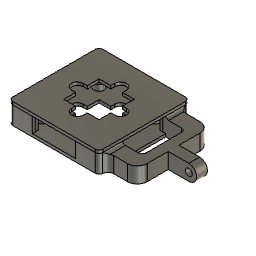
ArduCam Case v4 (Autodesk Fusion 360 design; units mm, degrees)
Autodesk Fusion 360 part; units mm, degrees
sketch "Base" plane through (0, 0, 0) normal (0, 0, 1) x (1, 0, 0)
  circle A0 centre (14.4, -14.4) radius 1.5
  circle A1 centre (-14.4, -14.4) radius 1.5
  circle A2 centre (-14.4, 14.4) radius 1.5
  circle A3 centre (14.4, 14.4) radius 1.5
  line L0 (18, 20) -> (-18, 20)
  line L1 (-20, 18) -> (-20, -18)
  line L2 (-18, -20) -> (18, -20)
  line L3 (20, -18) -> (20, 18)
  line L4 (19.5, -21.5) -> (-19.5, -21.5)
  line L5 (-21.5, -19.5) -> (-21.5, 19.5)
  line L6 (-19.5, 21.5) -> (19.5, 21.5)
  line L7 (21.5, -19.5) -> (21.5, 19.5)
  line L8 (21, 23) -> (-21, 23)
  line L9 (-23, 21) -> (-23, -21)
  line L10 (-21, -23) -> (21, -23)
  line L11 (23, 21) -> (23, -21)
  arc A4 (-18, 20) -> (-20, 18) centre (-18, 18) ccw
  arc A5 (-20, -18) -> (-18, -20) centre (-18, -18) ccw
  arc A6 (18, -20) -> (20, -18) centre (18, -18) ccw
  arc A7 (20, 18) -> (18, 20) centre (18, 18) ccw
  arc A8 (-19.5, 21.5) -> (-21.5, 19.5) centre (-19.5, 19.5) ccw
  arc A9 (-21.5, -19.5) -> (-19.5, -21.5) centre (-19.5, -19.5) ccw
  arc A10 (19.5, -21.5) -> (21.5, -19.5) centre (19.5, -19.5) ccw
  arc A11 (21.5, 19.5) -> (19.5, 21.5) centre (19.5, 19.5) ccw
  arc A12 (-21, 23) -> (-23, 21) centre (-21, 21) ccw
  arc A13 (-23, -21) -> (-21, -23) centre (-21, -21) ccw
  arc A14 (21, -23) -> (23, -21) centre (21, -21) ccw
  arc A15 (23, 21) -> (21, 23) centre (21, 21) ccw
  line L12 (9, -9) -> (-9, 9) construction
  line L13 (-9, -9) -> (9, 9) construction
  line L14 (9, 0) -> (11, 0)
  arc A16 (11, -3) -> (11, 3) centre (11, 0) ccw
  arc A17 (-3, -11) -> (3, -11) centre (0, -11) ccw
  arc A18 (-11, 3) -> (-11, -3) centre (-11, 0) ccw
  arc A19 (3, 11) -> (-3, 11) centre (0, 11) ccw
  line L15 (-9, 9) -> (-3, 9)
  line L16 (-3, 11) -> (-3, 9)
  line L17 (-9, 9) -> (-9, 3)
  line L18 (-9, 3) -> (-11, 3)
  line L19 (-11, -3) -> (-9, -3)
  line L20 (-9, -3) -> (-9, -9)
  line L21 (-9, -9) -> (-3, -9)
  line L22 (-3, -9) -> (-3, -11)
  line L23 (3, -11) -> (3, -9)
  line L24 (9, -3) -> (11, -3)
  line L25 (11, 3) -> (9, 3)
  line L26 (9, 3) -> (9, 9)
  line L27 (3, 9) -> (3, 11)
  line L28 (3, 9) -> (9, 9)
  line L29 (9, -9) -> (3, -9)
  line L30 (9, -9) -> (9, -3)
  circle A20 centre (14.4, 14.4) radius 2.5
  circle A21 centre (-14.4, 14.4) radius 2.5
  circle A22 centre (-14.4, -14.4) radius 2.5
  circle A23 centre (14.4, -14.4) radius 2.5
  line L31 (-23, -11) -> (-20, -11)
  line L32 (-20, 11) -> (-23, 11)
  line L33 (20, 11) -> (23, 11)
  line L34 (20, -11) -> (23, -11)
  line L35 (-11, 20) -> (-11, 23)
  line L36 (11, 20) -> (11, 23)
  line L37 (11, -20) -> (11, -23)
  line L38 (-11, -20) -> (-11, -23)
  circle A24 centre (-14.4, -14.4) radius 1.4
  circle A25 centre (14.4, -14.4) radius 1.4
  circle A26 centre (14.4, 14.4) radius 1.4
  circle A27 centre (-14.4, 14.4) radius 1.4
  point P0 (21.5, -21.5)
  point P1 (-21.5, -21.5)
  point P2 (-21.5, 21.5)
  point P3 (21.5, 21.5)
  dimension "d3" = 28.8
  dimension "d4" = 28.8
  dimension "d5" = 28.8
  dimension "d6" = 3
  dimension "d7" = 3
  dimension "d8" = 3
  dimension "d9" = 3
  dimension "d10" = 43
  dimension "d11" = 43
  dimension "d12" = 43
  dimension "d13" = 2
  dimension "d14" = 2
  dimension "d15" = 2
  dimension "d16" = 5
  dimension "d17" = 5
  dimension "d18" = 5
  dimension "d19" = 5
  dimension "d71" = 2.8
  dimension "d72" = 2.8
  dimension "d73" = 2.8
  dimension "d74" = 2.8
  constraint perpendicular L0 L1
  constraint perpendicular L1 L2
  constraint perpendicular L0 L3
  constraint perpendicular L4 L5
  constraint perpendicular L5 L6
  constraint perpendicular L5 L8
  constraint perpendicular L8 L9
  constraint perpendicular L9 L10
  constraint perpendicular L10 L11
  constraint tangent L0 A4
  constraint tangent L1 A4
  constraint tangent L1 A5
  constraint tangent L2 A5
  constraint equal A4 A5
  constraint tangent L2 A6
  constraint tangent L3 A6
  constraint equal A4 A6
  constraint tangent L0 A7
  constraint tangent L3 A7
  constraint equal A4 A7
  constraint coincident P2 L5
  constraint coincident P2 L6
  constraint tangent L5 A8
  constraint tangent L6 A8
  constraint coincident P1 L4
  constraint coincident P1 L5
  constraint tangent L4 A9
  constraint tangent L5 A9
  constraint equal A8 A9
  constraint coincident P0 L4
  constraint coincident P0 L7
  constraint tangent L4 A10
  constraint tangent L7 A10
  constraint equal A8 A10
  constraint coincident P3 L6
  constraint coincident P3 L7
  constraint tangent L6 A11
  constraint tangent L7 A11
  constraint equal A8 A11
  constraint tangent L8 A12
  constraint tangent L9 A12
  constraint tangent L9 A13
  constraint tangent L10 A13
  constraint equal A12 A13
  constraint tangent L10 A14
  constraint tangent L11 A14
  constraint equal A12 A14
  constraint tangent L8 A15
  constraint tangent L11 A15
  constraint equal A12 A15
  constraint coincident L12 origin
  constraint coincident L13 origin
  constraint coincident L14.end A16.centre
  constraint tangent A19 L16
  constraint tangent A18 L18
  constraint tangent A18 L19
  constraint tangent A17 L22
  constraint tangent A17 L23
  constraint tangent A16 L24
  constraint tangent A16 L25
  constraint tangent A19 L27
  constraint perpendicular L27 L28
  constraint perpendicular L23 L29
  constraint perpendicular L29 L30
  constraint concentric A3 A20
  constraint concentric A2 A21
  constraint concentric A1 A22
  constraint concentric A0 A23
  constraint coincident L9 L31.start
  constraint coincident L1 L31.end
  constraint perpendicular L1 L31
  constraint coincident L1 L32.start
  constraint coincident L9 L32.end
  constraint perpendicular L9 L32
  constraint coincident L3 L33.start
  constraint coincident L11 L33.end
  constraint perpendicular L11 L33
  constraint coincident L3 L34.start
  constraint coincident L11 L34.end
  constraint perpendicular L11 L34
  constraint coincident L0 L35.start
  constraint coincident L8 L35.end
  constraint perpendicular L8 L35
  constraint coincident L0 L36.start
  constraint coincident L8 L36.end
  constraint perpendicular L8 L36
  constraint coincident L2 L37.start
  constraint coincident L10 L37.end
  constraint perpendicular L10 L37
  constraint coincident L2 L38.start
  constraint coincident L10 L38.end
  constraint perpendicular L10 L38
  constraint concentric A1 A24
  constraint concentric A0 A25
  constraint concentric A3 A26
  constraint concentric A21 A27
  measures "d3" distance of A0.centre A3.centre
  measures "d4" distance of A2.centre A3.centre
  measures "d5" distance of A1.centre A2.centre
  measures "d6" diameter of A0
  measures "d7" diameter of A1
  measures "d8" diameter of A2
  measures "d9" diameter of A3
  measures "d10" distance of P0 P1
  measures "d11" distance of P1 P2
  measures "d12" distance of P2 P3
  measures "d13" radius of A4
  measures "d14" radius of A8
  measures "d15" radius of A12
  measures "d16" diameter of A20
  measures "d17" diameter of A21
  measures "d18" diameter of A22
  measures "d19" diameter of A23
  measures "d71" diameter of A24
  measures "d72" diameter of A25
  measures "d73" diameter of A26
  measures "d74" diameter of A27
extrude "Extrude1" add sketch "Base" along normal blind 1.5 contours A0 | A1 | A2 | A3 | L0 L1 L2 L3 A4 A5 A6 A7 | L0 L3 L6 L7 A7 A11 L33 L36 | L0 L6 L35 L36 | L0 L1 L5 L6 A4 A8 L32 L35 | L6 L7 L8 L11 A11 A15 L33 L36 | L6 L8 L35 L36 | L3 L7 L33 L34 | L5 L6 L8 L9 A8 A12 L32 L35 | L2 L3 L4 L7 A6 A10 L34 L37 | L7 L11 L33 L34 | L4 L7 L10 L11 A10 A14 L34 L37 | L1 L5 L31 L32 | L1 L2 L4 L5 A5 A9 L31 L38 | L5 L9 L31 L32 | L2 L4 L37 L38 | L4 L5 L9 L10 A9 A13 L31 L38 | L4 L10 L37 L38 | A20 | A21 | A22 | A23 | A24 | A25 | A26 | A27 makes body 1
extrude "Extrude2" add sketch "Base" along normal blind 3 from surface at 1.5 contours A20 | A21 | A22 | A23 bodies 1
extrude "Extrude3" add 4 faces at (-15.2598, 14.4745, 1.5) (-15.2598, -14.3255, 1.5) (13.5402, -14.3255, 1.5) (14.15, 13.967, 1.5) along direction (0, 0, 1) blind 6 on bodies 1 bodies 1
extrude "Extrude4" add sketch "Base" along normal blind 3 from surface at 7.5 separate body contours A0 | A1 | A2 | A3 | A20 | A21 | A22 | A23 | A24 | A25 | A26 | A27 makes body 2 at (-11.9124, -14.6489, 8.5) makes body 3 at (16.8876, -14.6489, 8.5) makes body 4 at (-11.9124, 14.1511, 8.5) makes body 5 at (16.8876, 14.1511, 8.5)
extrude "Extrude5" add sketch "Base" along normal blind 9 from surface at 1.5 contours L6 L7 L8 L11 A11 A15 L33 L36 | L5 L6 L8 L9 A8 A12 L32 L35 | L4 L7 L10 L11 A10 A14 L34 L37 | L4 L5 L9 L10 A9 A13 L31 L38 bodies 1
extrude "Extrude6" add sketch "Base" along normal blind 1.5 from surface at 10.5 contours A0 | A1 | A2 | A3 | L0 L1 L2 L3 A4 A5 A6 A7 | L0 L3 L6 L7 A7 A11 L33 L36 | L0 L6 L35 L36 | L0 L1 L5 L6 A4 A8 L32 L35 | L3 L7 L33 L34 | L2 L3 L4 L7 A6 A10 L34 L37 | L1 L5 L31 L32 | L1 L2 L4 L5 A5 A9 L31 L38 | L2 L4 L37 L38 | A20 | A21 | A22 | A23 | A24 | A25 | A26 | A27 bodies 2 3 4 5
extrude "Extrude7" add sketch "Base" along normal blind 1.5 from surface at 10.5 contours L6 L7 L8 L11 A11 A15 L33 L36 | L6 L8 L35 L36 | L5 L6 L8 L9 A8 A12 L32 L35 | L7 L11 L33 L34 | L4 L7 L10 L11 A10 A14 L34 L37 | L5 L9 L31 L32 | L4 L5 L9 L10 A9 A13 L31 L38 | L4 L10 L37 L38 bodies 2
extrude "Extrude8" add sketch "Base" along normal blind 9 from surface at 1.5 contours L0 L3 L6 L7 A7 A11 L33 L36 | L0 L1 L5 L6 A4 A8 L32 L35 | L2 L3 L4 L7 A6 A10 L34 L37 | L1 L2 L4 L5 A5 A9 L31 L38 bodies 2
chamfer "Chamfer2" distance 0.5 angle 45 4 edges at (13.0015, -14.9424, 7.5) (13.0015, 13.8576, 7.5) (-15.7985, -14.9424, 7.5) (-15.7985, 13.8576, 7.5) on bodies 1
sketch "Sketch2" plane through (0, 0, 0) normal (0, 1, 0) x (1, 0, 0)
  line L0 (23, -10.5) -> (23, 0)
  line L1 (23, 0) -> (33, 0)
  line L2 (33, 0) -> (33, -10.5)
  line L3 (33, -10.5) -> (23, -10.5)
  line L4 (33, 0) -> (33, -8)
  line L5 (33, -8) -> (43.5, -8)
  line L6 (33, 0) -> (43.5, 0)
  arc A0 (43.5, -8) -> (43.5, 0) centre (43.5, -4) ccw
  circle A1 centre (43.5, -4) radius 1.75
  dimension "d42" = 3.5
  constraint vertical L0
  constraint perpendicular L0 L1
  constraint perpendicular L1 L2
  constraint perpendicular L0 L3
  constraint coincident L2 L4.end
  constraint perpendicular L4 L5
  constraint perpendicular L4 L6
  constraint tangent L6 A0
  constraint tangent L5 A0
  constraint concentric A0 A1
  measures "d42" diameter of A1
extrude "Extrude9" add sketch "Sketch2" along normal mid plane 5.5 separate body contours L2 L4 L5 L6 A0 makes body 6
extrude "Extrude18" cut sketch "Base" along normal blind 5 from surface at 4.5 contours A0 | A1 | A2 | A3 bodies 1
extrude "Extrude10" add sketch "Sketch2" along normal blind 7.5 from surface at 11 contours L0 L1 L2 L3 L4 bodies 1
extrude "Extrude11" add sketch "Sketch2" against normal blind 7.5 from surface at -11 contours L0 L1 L2 L3 L4 bodies 1
move_body "Move1" bodies 6 to x (1, 0, 0) y (0, 1, 0) z (0, 0, 1) at (5, 0, 0)
sketch "Sketch3" plane through (0, 0, 0) normal (0, 1, 0) x (-1, 0, 0)
  line L0 (-38, 8) -> (-38, 0)
  line L1 (-38, 0) -> (-33, 0)
  line L2 (-33, 0) -> (-33, 8)
  line L3 (-33, 8) -> (-38, 8)
  constraint vertical L0
  constraint perpendicular L0 L1
  constraint perpendicular L1 L2
  constraint perpendicular L2 L3
extrude "Extrude12" add sketch "Sketch3" along normal mid plane 37 bodies 1 6
sketch "Sketch4" plane through (0, 0, 0) normal (0, 1, 0) x (1, 0, 0)
  line L0 (38, 0) -> (38, -8)
  line L1 (38, -8) -> (23, -10.5)
  line L2 (23, -10.5) -> (23, 0)
  line L3 (23, 0) -> (38, 0)
  line L4 (33, 0) -> (33, -8.8333)
  constraint vertical L0
  constraint parallel L0 L2
  constraint perpendicular L0 L3
  constraint coincident L3 L4.start
  constraint coincident L1 L4.end
  constraint perpendicular L3 L4
chamfer "Chamfer1" distance 2.5 angle 45 2 edges at (33, -14.75, 10.5) (33, 14.75, 10.5) on bodies 1
fillet "Fillet1" radius 5 2 edges at (38, -18.5, 4) (38, 18.5, 4) on bodies 1
sketch "Sketch5" plane through (0, 18.5, 0) normal (0, 1, 0) x (-1, 0, 0)
  line L0 (-33, 8) -> (-33, 0)
  line L1 (-33, 0) -> (-23, 0)
  line L2 (-23, 0) -> (-23, 10.5)
  line L3 (-23, 10.5) -> (-30.5, 10.5)
  line L4 (-30.5, 10.5) -> (-33, 8)
  line L5 (-33, 8) -> (-23, 8)
  line L6 (-23, 10.5) -> (-23, 8)
  line L7 (-23, 10.5) -> (-33, 10.5)
  line L8 (-33, 10.5) -> (-33, 8)
  constraint coincident L0.start L4.end
  constraint coincident L2 L5.end
  constraint perpendicular L2 L5
  constraint coincident L2.end L3.start
  constraint perpendicular L6 L7
  constraint perpendicular L5 L8
extrude "Extrude13" cut sketch "Sketch5" against normal blind 61 contours L2 L3 L4 L5 L6 L7 bodies 1
extrude "Extrude14" add sketch "Base" against normal blind 1.35 from surface at 7.5 contours A20 | A21 | A22 | A23 bodies 2
extrude "Extrude15" cut 1 faces at (0.0747, -19.9972, 12) along direction (0, 0, -1) blind 1.35 on bodies 2 bodies 2
extrude "Extrude16" add 1 faces at (-18.9972, -0.0747, 10.5) along direction (0, 0, -1) blind 1.35 on bodies 2 bodies 2
extrude "Extrude17" cut 4 faces at (22.5, 17.1667, 10.5) (22.5, -17.1667, 10.5) (-17.1667, -22.5, 10.5) (-17.1667, 22.5, 10.5) along direction (0, 0, -1) blind 1.35 on bodies 1 bodies 1
fillet "Fillet3" radius 1.5 2 edges at (23, -14.75, 8) (23, 14.75, 8) on bodies 1
fillet "Fillet4" radius 3 2 edges at (23, 18.5, 4.575) (23, -18.5, 4.575) on bodies 1
fillet "Fillet5" radius 2 2 edges at (33, 11, 4) (33, -11, 4) on bodies 1
copy_body "CopyPasteBodies1" bodies 1 makes body 7
copy_body "Body->Comp1" bodies 7 removing the originals makes body 8 in component "Bare Camera Case"
copy_body "CopyPasteBodies1'" bodies 2 makes body 9 in component "Bare Camera Case"
sketch "Sketch1" plane through (0, 0, 0) normal (0, 0, 1) x (1, 0, 0) in component "Bare Camera Case"
  line L0 (11, 20) -> (11, 23)
  circle A0 centre (14.4, -14.4) radius 1.5
  line L1 (23, 21) -> (23, -21)
  line L2 (9, -9) -> (9, -3)
  line L3 (3, -11) -> (3, -9)
  line L4 (20, -11) -> (23, -11)
  line L5 (3, 9) -> (3, 11)
  line L6 (-9, -9) -> (9, 9) construction
  line L7 (9, 3) -> (9, 9)
  line L8 (-21, -23) -> (21, -23)
  line L9 (3, 9) -> (9, 9)
  line L10 (11, -20) -> (11, -23)
  arc A1 (18, -20) -> (20, -18) centre (18, -18) ccw
  circle A2 centre (14.4, 14.4) radius 2.5
  circle A3 centre (14.4, -14.4) radius 1.4
  circle A4 centre (14.4, 14.4) radius 1.5
  line L11 (-11, -3) -> (-9, -3)
  line L12 (-21.5, -19.5) -> (-21.5, 19.5)
  arc A5 (-3, -11) -> (3, -11) centre (0, -11) ccw
  line L13 (21, 23) -> (-21, 23)
  line L14 (-19.5, 21.5) -> (19.5, 21.5)
  line L15 (18, 20) -> (-18, 20)
  arc A6 (3, 11) -> (-3, 11) centre (0, 11) ccw
  line L16 (9, 0) -> (11, 0)
  line L17 (-23, -11) -> (-20, -11)
  arc A7 (-19.5, 21.5) -> (-21.5, 19.5) centre (-19.5, 19.5) ccw
  line L18 (-20, 18) -> (-20, -18)
  line L19 (19.5, -21.5) -> (-19.5, -21.5)
  arc A8 (-18, 20) -> (-20, 18) centre (-18, 18) ccw
  line L20 (-18, -20) -> (18, -20)
  line L21 (9, -9) -> (-9, 9) construction
  arc A9 (11, -3) -> (11, 3) centre (11, 0) ccw
  line L22 (-20, 11) -> (-23, 11)
  circle A10 centre (-14.4, 14.4) radius 1.5
  circle A11 centre (-14.4, -14.4) radius 2.5
  line L23 (-3, 11) -> (-3, 9)
  arc A12 (23, 21) -> (21, 23) centre (21, 21) ccw
  arc A13 (-21.5, -19.5) -> (-19.5, -21.5) centre (-19.5, -19.5) ccw
  circle A14 centre (-14.4, -14.4) radius 1.4
  circle A15 centre (-14.4, -14.4) radius 1.5
  line L24 (-11, -20) -> (-11, -23)
  line L25 (-23, 21) -> (-23, -21)
  line L26 (-9, 3) -> (-11, 3)
  line L27 (-9, -3) -> (-9, -9)
  arc A16 (-20, -18) -> (-18, -20) centre (-18, -18) ccw
  arc A17 (-23, -21) -> (-21, -23) centre (-21, -21) ccw
  line L28 (-3, -9) -> (-3, -11)
  circle A18 centre (-14.4, 14.4) radius 2.5
  line L29 (-9, -9) -> (-3, -9)
  circle A19 centre (-14.4, 14.4) radius 1.4
  arc A20 (-11, 3) -> (-11, -3) centre (-11, 0) ccw
  line L30 (-9, 9) -> (-3, 9)
  arc A21 (-21, 23) -> (-23, 21) centre (-21, 21) ccw
  line L31 (-9, 9) -> (-9, 3)
  line L32 (-11, 20) -> (-11, 23)
  arc A22 (21.5, 19.5) -> (19.5, 21.5) centre (19.5, 19.5) ccw
  line L33 (9, -9) -> (3, -9)
  arc A23 (20, 18) -> (18, 20) centre (18, 18) ccw
  line L34 (20, 11) -> (23, 11)
  arc A24 (19.5, -21.5) -> (21.5, -19.5) centre (19.5, -19.5) ccw
  arc A25 (21, -23) -> (23, -21) centre (21, -21) ccw
  line L35 (9, -3) -> (11, -3)
  circle A26 centre (14.4, 14.4) radius 1.4
  line L36 (20, -18) -> (20, 18)
  line L37 (11, 3) -> (9, 3)
  line L38 (21.5, -19.5) -> (21.5, 19.5)
  circle A27 centre (14.4, -14.4) radius 2.5
  line L39 (30, 30) -> (-30, 30)
  line L40 (-30, 30) -> (-30, -30)
  line L41 (-30, -30) -> (30, -30)
  line L42 (30, -30) -> (30, 30)
  line L43 (30, 30) -> (-30, -30) construction
  line L44 (-30, 30) -> (30, -30) construction
  line L45 (65, 35) -> (-65, 35)
  line L46 (-65, 35) -> (-65, -35)
  line L47 (-65, -35) -> (65, -35)
  line L48 (65, -35) -> (65, 35)
  line L49 (65, 35) -> (-65, -35) construction
  line L50 (-65, 35) -> (65, -35) construction
  point P0 (-21.5, 21.5)
  point P1 (-21.5, -21.5)
  point P2 (21.5, 21.5)
  point P3 (21.5, -21.5)
  dimension "d78" = 28.8
  dimension "d79" = 28.8
  dimension "d80" = 28.8
  dimension "d81" = 3
  dimension "d82" = 3
  dimension "d83" = 3
  dimension "d84" = 3
  dimension "d85" = 43
  dimension "d86" = 43
  dimension "d87" = 43
  dimension "d88" = 2
  dimension "d89" = 2
  dimension "d90" = 2
  dimension "d91" = 5
  dimension "d92" = 5
  dimension "d93" = 5
  dimension "d94" = 5
  dimension "d95" = 2.8
  dimension "d96" = 2.8
  dimension "d97" = 2.8
  dimension "d98" = 2.8
  constraint perpendicular L15 L18
  constraint perpendicular L18 L20
  constraint perpendicular L15 L36
  constraint perpendicular L12 L19
  constraint perpendicular L12 L14
  constraint perpendicular L12 L13
  constraint perpendicular L13 L25
  constraint perpendicular L8 L25
  constraint perpendicular L1 L8
  constraint tangent L15 A8
  constraint tangent L18 A8
  constraint tangent L18 A16
  constraint tangent L20 A16
  constraint equal A8 A16
  constraint tangent A1 L20
  constraint tangent A1 L36
  constraint equal A1 A8
  constraint tangent L15 A23
  constraint tangent A23 L36
  constraint equal A8 A23
  constraint coincident P0 L12
  constraint coincident P0 L14
  constraint tangent L12 A7
  constraint tangent L14 A7
  constraint coincident P1 L19
  constraint coincident P1 L12
  constraint tangent L19 A13
  constraint tangent L12 A13
  constraint equal A7 A13
  constraint coincident P3 L19
  constraint coincident P3 L38
  constraint tangent L19 A24
  constraint tangent A24 L38
  constraint equal A7 A24
  constraint coincident P2 L14
  constraint coincident P2 L38
  constraint tangent L14 A22
  constraint tangent A22 L38
  constraint equal A7 A22
  constraint tangent L13 A21
  constraint tangent L25 A21
  constraint tangent L25 A17
  constraint tangent L8 A17
  constraint equal A17 A21
  constraint tangent L8 A25
  constraint tangent L1 A25
  constraint equal A21 A25
  constraint tangent L13 A12
  constraint tangent L1 A12
  constraint equal A12 A21
  constraint coincident origin L21
  constraint coincident origin L6
  constraint coincident L16.end A9.centre
  constraint tangent A6 L23
  constraint tangent L26 A20
  constraint tangent L11 A20
  constraint tangent A5 L28
  constraint tangent L3 A5
  constraint tangent A9 L35
  constraint tangent A9 L37
  constraint tangent L5 A6
  constraint perpendicular L5 L9
  constraint perpendicular L3 L33
  constraint perpendicular L2 L33
  constraint concentric A2 A4
  constraint concentric A10 A18
  constraint concentric A11 A15
  constraint concentric A0 A27
  constraint coincident L17.start L25
  constraint coincident L17.end L18
  constraint perpendicular L17 L18
  constraint coincident L22.start L18
  constraint coincident L22.end L25
  constraint perpendicular L22 L25
  constraint coincident L34.start L36
  constraint coincident L34.end L1
  constraint perpendicular L1 L34
  constraint coincident L4.start L36
  constraint coincident L4.end L1
  constraint perpendicular L1 L4
  constraint coincident L32.start L15
  constraint coincident L32.end L13
  constraint perpendicular L13 L32
  constraint coincident L0.start L15
  constraint coincident L0.end L13
  constraint perpendicular L0 L13
  constraint coincident L10.start L20
  constraint coincident L10.end L8
  constraint perpendicular L8 L10
  constraint coincident L24.start L20
  constraint coincident L24.end L8
  constraint perpendicular L8 L24
  constraint concentric A14 A15
  constraint concentric A0 A3
  constraint concentric A4 A26
  constraint concentric A18 A19
  constraint horizontal L39
  constraint perpendicular L39 L40
  constraint parallel L39 L41
  constraint parallel L40 L42
  constraint coincident L43 origin
  constraint coincident L44 origin
  constraint horizontal L45
  constraint perpendicular L45 L46
  constraint parallel L45 L47
  constraint parallel L46 L48
  constraint coincident L49 origin
  constraint coincident L50 origin
  measures "d78" distance of A0.centre A2.centre
  measures "d79" distance of A10.centre A2.centre
  measures "d80" distance of A11.centre A10.centre
  measures "d81" diameter of A0
  measures "d82" diameter of A15
  measures "d83" diameter of A10
  measures "d84" diameter of A4
  measures "d85" distance of P1 P3
  measures "d86" distance of P0 P1
  measures "d87" distance of P0 P2
  measures "d88" radius of A8
  measures "d89" radius of A7
  measures "d90" radius of A21
  measures "d91" diameter of A2
  measures "d92" diameter of A18
  measures "d93" diameter of A11
  measures "d94" diameter of A27
  measures "d95" diameter of A14
  measures "d96" diameter of A3
  measures "d97" diameter of A26
  measures "d98" diameter of A19
extrude "Extrude1'" cut sketch "Sketch1" along normal blind 50 contours L39 L40 L41 L42 | L45 L46 L47 L48 bodies 8 in component "Bare Camera Case"
component "Bare Camera Case" placed x (1, 0, 0) y (0, 1, 0) z (0, 0, 1) at (0, 0, 0)
named bodies: "ArduCam Case (Front)", "ArduCam Case (Back)", "Front Piece", "Front Piece (1)", "Back Piece"
